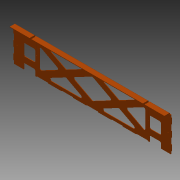
# Autodesk Inventor part: Brace
Saved by Autodesk Inventor 2014 (Build 180170000, 170)
## iProperties
Created: 2014-01-11
Part Number: Brace
Material: Aluminum 6061
Document SubType Name: Sheet Metal
Designer: Alex
Density: 2.71 g/cm^3
Sheet Metal Rule: Default
Appearance: Smooth - Light Orange
Mass: 689.694 g
Surface Area: 2287.02 cm^2
Volume: 254.5 cm^3
Author: Alex
Autodesk Inventor part; units mm, degrees
ref_plane "YZ Plane" through (0, 0, 0) normal (1, 0, 0) x (0, 1, 0)
ref_plane "XZ Plane" through (0, 0, 0) normal (0, 1, 0) x (-1, 0, 0)
ref_plane "XY Plane" through (0, 0, 0) normal (0, 0, 1) x (1, 0, 0)
sketch "Sketch1" plane through (0, 0, 0) normal (0, 0, 1) x (1, 0, 0)
  line L0 (-361.4596, 78.6852) -> (326.3724, 78.6852)
  line L1 (326.3724, -76.0008) -> (-361.4596, -76.0008)
  line L2 (328.6584, 63.6992) -> (326.3724, 63.6992)
  line L3 (326.3724, 63.6992) -> (326.3724, 38.2992)
  line L4 (326.3724, 38.2992) -> (328.6584, 38.2992)
  line L5 (328.6584, 38.2992) -> (328.6584, 63.6992)
  line L6 (326.3724, -12.5008) -> (328.6584, -12.5008)
  line L7 (328.6584, -12.5008) -> (328.6584, 12.8992)
  line L8 (328.6584, 12.8992) -> (326.3724, 12.8992)
  line L9 (326.3724, 12.8992) -> (326.3724, -12.5008)
  line L10 (328.6584, -37.9008) -> (326.3724, -37.9008)
  line L11 (326.3724, -37.9008) -> (326.3724, -63.3008)
  line L12 (326.3724, -63.3008) -> (328.6584, -63.3008)
  line L13 (328.6584, -63.3008) -> (328.6584, -37.9008)
  line L14 (-361.4596, 78.6852) -> (-361.4596, 63.6992)
  line L15 (-361.4596, 38.2992) -> (-361.4596, -76.0008)
  line L16 (326.3724, 78.6852) -> (326.3724, 63.6992)
  line L17 (326.3724, 38.2992) -> (326.3724, -76.0008)
  line L18 (328.6584, 63.6992) -> (328.6584, 38.2992)
  line L19 (328.6584, 12.8992) -> (328.6584, -12.5008)
  line L20 (328.6584, -37.9008) -> (328.6584, -63.3008)
  line L21 (-363.7456, 63.6992) -> (-361.4596, 63.6992)
  line L22 (-361.4596, 38.2992) -> (-363.7456, 38.2992)
  line L23 (-363.7456, 38.2992) -> (-363.7456, 63.6992)
  line L24 (-361.4596, -12.5008) -> (-363.7456, -12.5008)
  line L25 (-363.7456, -12.5008) -> (-363.7456, 12.8992)
  line L26 (-363.7456, 12.8992) -> (-361.4596, 12.8992)
  line L27 (-363.7456, -37.9008) -> (-361.4596, -37.9008)
  line L28 (-361.4596, -63.3008) -> (-363.7456, -63.3008)
  line L29 (-363.7456, -63.3008) -> (-363.7456, -37.9008)
  line L30 (-361.4596, -37.9008) -> (-361.4596, -63.3008)
  line L31 (-361.4596, -12.5008) -> (-361.4596, 12.8992)
  line L32 (-363.7456, 12.8992) -> (-361.4596, 12.8992)
  line L33 (-361.4596, 12.8992) -> (-361.4596, -12.5008)
  line L34 (-361.4596, -12.5008) -> (-363.7456, -12.5008)
  line L35 (-363.7456, -12.5008) -> (-363.7456, 12.8992)
  line L36 (-363.7456, -37.9008) -> (-361.4596, -37.9008)
  line L37 (-361.4596, -37.9008) -> (-361.4596, -63.3008)
  line L38 (-361.4596, -63.3008) -> (-363.7456, -63.3008)
  line L39 (-363.7456, -63.3008) -> (-363.7456, -37.9008)
  line L40 (-262.1456, 74.3672) -> (-262.1456, -76.0008)
  line L41 (227.0584, -76.0008) -> (227.0584, 76.3992)
  line L42 (-262.1456, -76.0008) -> (-211.3456, -76.0008)
  line L43 (-211.3456, -76.0008) -> (-211.3456, -73.4608)
  line L44 (-211.3456, -73.4608) -> (-262.1456, -73.4608)
  line L45 (-262.1456, -73.4608) -> (-262.1456, -76.0008)
  line L46 (-102.3161, -76.0008) -> (-102.3161, -73.4608)
  line L47 (-102.3161, -73.4608) -> (-153.1161, -73.4608)
  line L48 (-153.1161, -73.4608) -> (-153.1161, -76.0008)
  line L49 (6.7134, -76.0008) -> (6.7134, -73.4608)
  line L50 (6.7134, -73.4608) -> (-44.0866, -73.4608)
  line L51 (-44.0866, -73.4608) -> (-44.0866, -76.0008)
  line L52 (115.7429, -76.0008) -> (115.7429, -73.4608)
  line L53 (115.7429, -73.4608) -> (64.9429, -73.4608)
  line L54 (64.9429, -73.4608) -> (64.9429, -76.0008)
  line L55 (224.7723, -76.0008) -> (224.7723, -73.4608)
  line L56 (224.7723, -73.4608) -> (173.9723, -73.4608)
  line L57 (173.9723, -73.4608) -> (173.9723, -76.0008)
  line L58 (-153.1161, -76.0008) -> (-102.3161, -76.0008)
  line L59 (-44.0866, -76.0008) -> (6.7134, -76.0008)
  line L60 (64.9429, -76.0008) -> (115.7429, -76.0008)
  line L61 (173.9723, -76.0008) -> (224.7723, -76.0008)
  line L62 (-361.4596, 78.6852) -> (-356.3796, 78.6852)
  line L63 (-356.3796, 78.6852) -> (-356.3796, 74.1132)
  line L64 (-356.3796, 74.1132) -> (-361.4596, 74.1132)
  line L65 (-361.4596, 74.1132) -> (-361.4596, 78.6852)
  line L66 (326.3724, 78.6852) -> (321.2924, 78.6852)
  line L67 (321.2924, 78.6852) -> (321.2924, 74.1132)
  line L68 (321.2924, 74.1132) -> (326.3724, 74.1132)
  line L69 (326.3724, 74.1132) -> (326.3724, 78.6852)
  point P0 (0, 0)
  point P1 (-362.6026, 63.6992)
  dimension "d0" = 687.832
  dimension "d3" = 2.286
  dimension "d4" = 25.4
  dimension "d5" = 14.986
  dimension "d6" = 25.4
  dimension "d7" = 2.286
  dimension "d8" = 25.4
  dimension "d9" = 2.286
  dimension "d10" = 25.4
  dimension "d11" = 25.4
  dimension "d12" = 2.286
  dimension "d13" = 2.286
  dimension "d16" = 50.8
  dimension "d17" = 2.54
  dimension "d21" = 109.0295
  dimension "d84" = 5.08
  dimension "d85" = 5.08
  dimension "d90" = 4.572
  dimension "d91" = 4.572
  measures "d0" distance of L1.start L1.end
  measures "d3" distance of L4.end L3.end
  measures "d4" distance of L3.end L2.end
  measures "d5" distance between parallel lines of L0 L2
  measures "d6" distance of L8.end L6.start
  measures "d7" distance of L7.end L8.end
  measures "d8" distance from line of L3.end L8
  measures "d9" distance of L12.end L11.end
  measures "d10" distance of L11.end L10.end
  measures "d11" distance between parallel lines of L6 L10
  measures "d12" distance of L24.start L25.start
  measures "d13" distance of L15.start L23.start
  measures "d16" distance of L44.end L43.end
  measures "d17" distance of L43.end L42.end
  measures "d21" distance of L44.end L48.start
  measures "d84" distance of L63.end L64.end
  measures "d85" distance of L68.end L67.end
  measures "d90" distance between parallel lines of L62 L64
  measures "d91" distance between parallel lines of L0 L68
extrude "Plate1" add sketch "Sketch1" along normal blind 2.286 contours L0 L67 L68 L16 L3 L17 L9 L11 L1 L55 L56 L57 L52 L53 L54 L49 L50 L51 L46 L47 L48 L43 L44 L40 L15 L22 L23 L21 L14 L64 L63 | L2 L5 L4 L3 | L15 L24 L25 L26 | L8 L7 L6 L9 | L15 L28 L29 L27 | L10 L13 L12 L11
sketch "Sketch3" plane through (0, 0, 2.286) normal (0, 0, 1) x (1, 0, 0)
  line L0 (328.6584, 12.8992) -> (328.6584, -12.5008) projected
  line L1 (-356.3796, 78.6852) -> (321.2924, 78.6852) projected
  line L2 (-363.7456, -12.5008) -> (-363.7456, 12.8992) projected
  line L3 (-264.4316, 78.6852) -> (-262.1456, 78.6852)
  line L4 (-262.1456, 78.6852) -> (-262.1456, 2.4852)
  line L5 (-262.1456, 2.4852) -> (-264.4316, 2.4852)
  line L6 (-264.4316, 2.4852) -> (-264.4316, 78.6852)
  line L7 (227.0584, 78.6852) -> (229.3444, 78.6852)
  line L8 (229.3444, 78.6852) -> (229.3444, 2.4852)
  line L9 (229.3444, 2.4852) -> (227.0584, 2.4852)
  line L10 (227.0584, 2.4852) -> (227.0584, 78.6852)
  line L11 (-264.4316, 78.6852) -> (-269.5116, 78.6852)
  line L12 (-269.5116, 78.6852) -> (-269.5116, 74.1132)
  line L13 (-269.5116, 74.1132) -> (-264.4316, 74.1132)
  line L14 (-264.4316, 74.1132) -> (-264.4316, 78.6852)
  line L15 (229.3444, 78.6852) -> (234.4244, 78.6852)
  line L16 (234.4244, 78.6852) -> (234.4244, 74.1132)
  line L17 (234.4244, 74.1132) -> (229.3444, 74.1132)
  line L18 (229.3444, 74.1132) -> (229.3444, 78.6852)
  point P0 (326.3724, 78.6852)
  point P1 (-361.4596, 78.6852)
  point P2 (0, 0)
  dimension "d26" = 2.286
  dimension "d27" = 76.2
  dimension "d28" = 101.6
  dimension "d29" = 2.286
  dimension "d30" = 76.2
  dimension "d31" = 101.6
  dimension "d86" = 5.08
  dimension "d87" = 5.08
  dimension "d88" = 4.572
  dimension "d89" = 4.572
  constraints: 32 end point, 8 parallel, 4 horizontal, 4 perpendicular, 2 point on line
  measures "d26" distance of L4.end L5.end
  measures "d27" distance of L3.end L4.end
  measures "d28" distance between parallel lines of L2 L4
  measures "d29" distance of L8.end L9.end
  measures "d30" distance of L7.end L8.end
  measures "d31" distance between parallel lines of L0 L10
  measures "d86" distance of L13.end L12.end
  measures "d87" distance of L16.end L17.end
  measures "d88" distance between parallel lines of L1 L13
  measures "d89" distance between parallel lines of L1 L17
extrude "Cut2" cut sketch "Sketch3" against normal blind 2.286
sketch "Sketch4" plane through (0, 0, 2.286) normal (0, 0, 1) x (1, 0, 0)
  line L0 (229.3444, 74.1132) -> (229.3444, 2.4852) projected
  line L1 (-264.4316, 2.4852) -> (-264.4316, 74.1132) projected
  line L2 (-262.1456, -76.0008) -> (-361.4596, -76.0008) projected
  line L3 (326.3724, -76.0008) -> (224.7723, -76.0008) projected
  line L4 (-267.6066, -76.0008) -> (-318.4066, -76.0008)
  line L5 (-318.4066, -76.0008) -> (-318.4066, 25.5992)
  line L6 (-318.4066, 25.5992) -> (-267.6066, 25.5992)
  line L7 (-267.6066, 25.5992) -> (-267.6066, -76.0008)
  line L8 (283.3194, -76.0008) -> (232.5194, -76.0008)
  line L9 (232.5194, -76.0008) -> (232.5194, 25.5992)
  line L10 (232.5194, 25.5992) -> (283.3194, 25.5992)
  line L11 (283.3194, 25.5992) -> (283.3194, -76.0008)
  point P0 (229.3444, 78.6852)
  point P1 (-264.4316, 78.6852)
  point P2 (0, 0)
  dimension "d34" = 50.8
  dimension "d35" = 101.6
  dimension "d37" = 3.175
  dimension "d38" = 50.8
  dimension "d40" = 3.175
  dimension "d41" = 101.6
  constraints: 16 end point, 4 parallel, 2 collinear, 2 horizontal, 2 perpendicular
  measures "d34" distance of L5.end L6.end
  measures "d35" distance between parallel lines of L6 L4
  measures "d37" distance between parallel lines of L7 L1
  measures "d38" distance of L9.end L10.end
  measures "d40" distance between parallel lines of L0 L9
  measures "d41" distance between parallel lines of L10 L8
extrude "Cut3" cut sketch "Sketch4" against normal blind 2.286
fillet "Corner Round1" radius 6.35 4 edges at (-318.4066, 25.5992, 1.143) (-267.6066, 25.5992, 1.143) (283.3194, 25.5992, 1.143) (232.5194, 25.5992, 1.143)
sketch "Sketch5" plane through (0, 0, 2.286) normal (0, 0, 1) x (1, 0, 0)
  line L0 (-267.6066, 19.2492) -> (-267.6066, -76.0008) projected
  arc A0 (-277.1316, -37.9008) -> (-270.7816, -31.5508) centre (-277.1316, -31.5508) ccw projected
  line L1 (-277.1316, -37.9008) -> (-340.6316, -37.9008) projected
  arc A1 (-346.9816, -31.5508) -> (-340.6316, -37.9008) centre (-340.6316, -31.5508) ccw projected
  line L2 (-318.4066, -76.0008) -> (-318.4066, 19.2492) projected
  arc A2 (-312.0566, 25.5992) -> (-318.4066, 19.2492) centre (-312.0566, 19.2492) ccw projected
  line L3 (-312.0566, 25.5992) -> (-273.9566, 25.5992) projected
  arc A3 (-267.6066, 19.2492) -> (-273.9566, 25.5992) centre (-273.9566, 19.2492) ccw projected
  line L4 (283.3194, 19.2492) -> (283.3194, -76.0008) projected
  arc A4 (305.5444, -37.9008) -> (311.8944, -31.5508) centre (305.5444, -31.5508) ccw projected
  line L5 (305.5444, -37.9008) -> (242.0444, -37.9008) projected
  arc A5 (235.6944, -31.5508) -> (242.0444, -37.9008) centre (242.0444, -31.5508) ccw projected
  line L6 (232.5194, -76.0008) -> (232.5194, 19.2492) projected
  arc A6 (238.8694, 25.5992) -> (232.5194, 19.2492) centre (238.8694, 19.2492) ccw projected
  line L7 (238.8694, 25.5992) -> (276.9694, 25.5992) projected
  arc A7 (283.3194, 19.2492) -> (276.9694, 25.5992) centre (276.9694, 19.2492) ccw projected
  line L8 (229.3444, 74.1132) -> (229.3444, 2.4852) projected
  line L9 (229.3444, 2.4852) -> (227.0584, 2.4852) projected
  line L10 (227.0584, 2.4852) -> (227.0584, 78.6852) projected
  line L11 (-262.1456, 78.6852) -> (227.0584, 78.6852) projected
  line L12 (-262.1456, 78.6852) -> (-262.1456, 2.4852) projected
  line L13 (-262.1456, 2.4852) -> (-264.4316, 2.4852) projected
  line L14 (-264.4316, 2.4852) -> (-264.4316, 74.1132) projected
  line L15 (-356.3796, 78.6852) -> (-269.5116, 78.6852) projected
  line L16 (-361.4596, 63.6992) -> (-361.4596, 74.1132) projected
  line L17 (-363.7456, 63.6992) -> (-361.4596, 63.6992) projected
  line L18 (-363.7456, 38.2992) -> (-363.7456, 63.6992) projected
  line L19 (-361.4596, 38.2992) -> (-363.7456, 38.2992) projected
  line L20 (-361.4596, 12.8992) -> (-361.4596, 38.2992) projected
  line L21 (-363.7456, 12.8992) -> (-361.4596, 12.8992) projected
  line L22 (-363.7456, -12.5008) -> (-363.7456, 12.8992) projected
  line L23 (-361.4596, -12.5008) -> (-363.7456, -12.5008) projected
  line L24 (-361.4596, -37.9008) -> (-361.4596, -12.5008) projected
  line L25 (-363.7456, -37.9008) -> (-361.4596, -37.9008) projected
  line L26 (-363.7456, -63.3008) -> (-363.7456, -37.9008) projected
  line L27 (-361.4596, -63.3008) -> (-363.7456, -63.3008) projected
  line L28 (-361.4596, -76.0008) -> (-361.4596, -63.3008) projected
  line L29 (-262.1456, -76.0008) -> (-361.4596, -76.0008) projected
  line L30 (-262.1456, -76.0008) -> (-262.1456, -73.4608) projected
  line L31 (-262.1456, -73.4608) -> (-211.3456, -73.4608) projected
  line L32 (-211.3456, -73.4608) -> (-211.3456, -76.0008) projected
  line L33 (-153.1161, -76.0008) -> (-211.3456, -76.0008) projected
  line L34 (-153.1161, -76.0008) -> (-153.1161, -73.4608) projected
  line L35 (-153.1161, -73.4608) -> (-102.3161, -73.4608) projected
  line L36 (-102.3161, -73.4608) -> (-102.3161, -76.0008) projected
  line L37 (-44.0866, -76.0008) -> (-102.3161, -76.0008) projected
  line L38 (-44.0866, -76.0008) -> (-44.0866, -73.4608) projected
  line L39 (-44.0866, -73.4608) -> (6.7134, -73.4608) projected
  line L40 (6.7134, -73.4608) -> (6.7134, -76.0008) projected
  line L41 (64.9429, -76.0008) -> (6.7134, -76.0008) projected
  line L42 (64.9429, -76.0008) -> (64.9429, -73.4608) projected
  line L43 (64.9429, -73.4608) -> (115.7429, -73.4608) projected
  line L44 (115.7429, -73.4608) -> (115.7429, -76.0008) projected
  line L45 (173.9723, -76.0008) -> (115.7429, -76.0008) projected
  line L46 (173.9723, -76.0008) -> (173.9723, -73.4608) projected
  line L47 (173.9723, -73.4608) -> (224.7723, -73.4608) projected
  line L48 (224.7723, -73.4608) -> (224.7723, -76.0008) projected
  line L49 (326.3724, -76.0008) -> (224.7723, -76.0008) projected
  line L50 (326.3724, -63.3008) -> (326.3724, -76.0008) projected
  line L51 (328.6584, -63.3008) -> (326.3724, -63.3008) projected
  line L52 (328.6584, -37.9008) -> (328.6584, -63.3008) projected
  line L53 (326.3724, -37.9008) -> (328.6584, -37.9008) projected
  line L54 (326.3724, -12.5008) -> (326.3724, -37.9008) projected
  line L55 (328.6584, -12.5008) -> (326.3724, -12.5008) projected
  line L56 (328.6584, 12.8992) -> (328.6584, -12.5008) projected
  line L57 (326.3724, 12.8992) -> (328.6584, 12.8992) projected
  line L58 (326.3724, 38.2992) -> (326.3724, 12.8992) projected
  line L59 (328.6584, 38.2992) -> (326.3724, 38.2992) projected
  line L60 (328.6584, 63.6992) -> (328.6584, 38.2992) projected
  line L61 (326.3724, 63.6992) -> (328.6584, 63.6992) projected
  line L62 (326.3724, -63.3008) -> (326.3724, 63.6992) projected
  line L63 (-356.3796, 78.6852) -> (-269.5116, 78.6852) projected
  point P0 (229.3444, 78.6852)
  point P1 (-264.4316, 78.6852)
  point P2 (-361.4596, 78.6852)
  point P3 (326.3724, 78.6852)
  point P4 (0, 0)
  constraints: 4 other
sketch "Sketch6" plane through (-262.1456, 76.3992, 0) normal (0, 1, 0) x (-1, 0, 0)
  line L0 (-489.204, 0) -> (0, 0)
  line L1 (0, 0) -> (0, 25.4)
  line L2 (0, 25.4) -> (-489.204, 25.4)
  line L3 (-489.204, 25.4) -> (-489.204, 0)
  constraints: 6 end point, 1 horizontal, 1 perpendicular, 1 vertical
edge flange "Flange1" height 25.4 angle 90 thickness 2.286 bend radius 2.286 thickness toward (0, 1, 0) relief straight relief width 2.286 relief depth 1.143 corner gap 2.286 corner form 0 edges at (-17.5436, 78.6852, 2.286) (277.8584, 78.6852, 2.286) (-312.9456, 78.6852, 2.286) wall of the first edge with corners at (227.0584, 76.3992, 0) (-262.1456, 76.3992, 0) (-262.1456, 76.3992, 25.4) (227.0584, 76.3992, 25.4)
bend "Bend1"
corner "Corner1"
sketch "Sketch7" plane through (0, 0, 2.286) normal (0, 0, 1) x (1, 0, 0)
  line L0 (-318.4066, -76.0008) -> (-361.4596, -76.0008)
  line L1 (-318.4066, -76.0008) -> (-318.4066, 19.2492)
  line L2 (-267.6066, 19.2492) -> (-267.6066, -76.0008)
  line L3 (232.5194, -76.0008) -> (224.7723, -76.0008)
  line L4 (232.5194, -76.0008) -> (232.5194, 19.2492)
  line L5 (283.3194, 19.2492) -> (283.3194, -76.0008)
  line L6 (232.5194, -25.2008) -> (283.3194, -25.2008)
  line L7 (283.3194, -25.2008) -> (283.3194, -50.6008)
  line L8 (283.3194, -50.6008) -> (232.5194, -50.6008)
  line L9 (232.5194, -50.6008) -> (232.5194, -25.2008)
  line L10 (-267.6066, -50.6008) -> (-318.4066, -50.6008)
  line L11 (-318.4066, -50.6008) -> (-318.4066, -25.2008)
  line L12 (-318.4066, -25.2008) -> (-267.6066, -25.2008)
  line L13 (-267.6066, -25.2008) -> (-267.6066, -50.6008)
  point P0 (0, 0)
  dimension "d55" = 25.4
  dimension "d56" = 25.4
  dimension "d57" = 25.4
  dimension "d58" = 25.4
  measures "d55" distance between parallel lines of L8 L3
  measures "d56" distance between parallel lines of L8 L6
  measures "d57" distance between parallel lines of L10 L0
  measures "d58" distance between parallel lines of L10 L12
sheet face with bend "Face2" sketch "Sketch7" thickness 2.286 toward (0, 0, -1) bend radius 2.286 relief straight relief width 2.286 relief depth 1.143
bend "Bend2"
fillet "Corner Round2" radius 6.35 8 edges at (-318.4066, -25.2008, 1.143) (-267.6066, -25.2008, 1.143) (283.3194, -25.2008, 1.143) (232.5194, -25.2008, 1.143) (283.3194, -50.6008, 1.143) (232.5194, -50.6008, 1.143) (-318.4066, -50.6008, 1.143) (-267.6066, -50.6008, 1.143)
sketch "Sketch8" plane through (0, 0, 2.286) normal (0, 0, 1) x (1, 0, 0)
  line L0 (227.0584, 2.4852) -> (227.0584, 74.1132) projected
  line L1 (227.0584, 74.1132) -> (-262.1456, 74.1132) projected
  line L2 (-262.1456, 74.1132) -> (-262.1456, 2.4852) projected
  line L3 (64.9429, -73.4608) -> (115.7429, -73.4608) projected
  line L4 (-249.4456, 61.4132) -> (214.3584, 61.4132)
  line L5 (214.3584, 61.4132) -> (214.3584, -60.7608)
  line L6 (214.3584, -60.7608) -> (-249.4456, -60.7608)
  line L7 (-249.4456, -60.7608) -> (-249.4456, 61.4132)
  line L8 (-17.5436, 61.4132) -> (214.3584, -60.7608)
  line L9 (214.3584, 61.4132) -> (-17.5436, -60.7608)
  line L10 (-249.4456, 61.4132) -> (-17.5436, -60.7608)
  line L11 (-17.5436, 61.4132) -> (-249.4456, -60.7608)
  line L12 (-222.1985, -60.7608) -> (-119.871, -6.8512)
  line L13 (-17.5436, -60.7608) -> (-133.4946, 0.3262)
  line L14 (-44.7906, -60.7608) -> (-147.1181, -6.8512)
  line L15 (-147.1181, -6.8512) -> (-249.4456, 47.0585)
  line L16 (-249.4456, -46.4061) -> (-133.4946, 14.6809)
  line L17 (9.7035, -60.7608) -> (-222.1985, 61.4132)
  line L18 (-119.871, -6.8512) -> (9.7035, 61.4132)
  line L19 (187.1114, -60.7608) -> (-31.1671, 54.2358)
  line L20 (214.3584, -46.4061) -> (9.7035, 61.4132)
  line L21 (217.3789, 48.6498) -> (9.7035, -60.7608)
  line L22 (187.1114, 61.4132) -> (-44.7906, -60.7608)
  line L23 (-222.1985, 61.4132) -> (-133.4946, 14.6809)
  line L24 (-133.4946, 14.6809) -> (-88.6639, 38.2992)
  line L25 (-44.7906, 61.4132) -> (-222.1985, 61.4132)
  line L26 (-249.4456, 47.0585) -> (-160.7416, 0.3262)
  line L27 (-160.7416, 0.3262) -> (-249.4456, -46.4061)
  line L28 (-222.1985, -60.7608) -> (-133.4946, -14.0285)
  line L29 (-133.4946, -14.0285) -> (-44.7906, -60.7608)
  line L30 (-44.7906, -60.7608) -> (-222.1985, -60.7608)
  line L31 (-17.5436, -46.4061) -> (71.1604, 0.3262)
  line L32 (71.1604, 0.3262) -> (-17.5436, 47.0585)
  line L33 (-106.2475, 0.3262) -> (-17.5436, 47.0585)
  line L34 (-106.2475, 0.3262) -> (-17.5436, -46.4061)
  line L35 (9.7035, -60.7608) -> (98.4074, -14.0285)
  line L36 (187.1114, -60.7608) -> (98.4074, -14.0285)
  line L37 (187.1114, -60.7608) -> (9.7035, -60.7608)
  line L38 (125.6545, 0.3262) -> (214.3584, -46.4061)
  line L39 (187.1114, 61.4132) -> (98.4074, 14.6809)
  line L40 (98.4074, 14.6809) -> (9.7035, 61.4132)
  line L41 (-44.7906, 61.4132) -> (-222.1985, 61.4132)
  line L42 (-88.6639, 38.2992) -> (-133.4946, 14.6809)
  line L43 (-133.4946, 14.6809) -> (-222.1985, 61.4132)
  line L44 (232.5194, -76.0008) -> (232.5194, -56.9508) projected
  line L45 (9.7035, 61.4132) -> (98.4074, 14.6809)
  line L46 (98.4074, 14.6809) -> (187.1114, 61.4132)
  line L47 (187.1114, 61.4132) -> (9.7035, 61.4132)
  line L48 (214.3584, 47.0585) -> (125.6545, 0.3262)
  line L49 (125.6545, 0.3262) -> (214.3584, -46.4061)
  line L50 (214.3584, -46.4061) -> (214.3584, 47.0585)
  line L51 (232.5194, -76.0008) -> (224.7723, -76.0008) projected
  line L52 (-133.4946, -14.0285) -> (-44.7906, -60.7608)
  line L53 (-44.7906, -60.7608) -> (-222.1985, -60.7608)
  line L54 (-222.1985, -60.7608) -> (-133.4946, -14.0285)
  line L55 (-133.4946, 14.6809) -> (-88.6639, 38.2992)
  line L56 (-44.7906, 61.4132) -> (-222.1985, 61.4132)
  line L57 (-222.1985, 61.4132) -> (-133.4946, 14.6809)
  line L58 (-361.4596, 38.2992) -> (-363.7456, 38.2992) projected
  line L59 (-133.4946, 14.6809) -> (-44.7906, 61.4132)
  line L60 (-44.7906, 61.4132) -> (-222.1985, 61.4132)
  point P0 (0, 0)
  point P1 (227.0584, 78.6852)
  point P2 (-262.1456, 78.6852)
  dimension "d65" = 12.7
  dimension "d66" = 12.7
  dimension "d67" = 12.7
  dimension "d68" = 12.7
  dimension "d69" = 12.7
  dimension "d71" = 231.902
  dimension "d72" = 463.804
  dimension "d73" = 231.902
  dimension "d74" = 12.7
  dimension "d75" = 12.7
  dimension "d76" = 12.7
  dimension "d77" = 12.7
  dimension "d78" = 12.7
  dimension "d79" = 12.7
  constraints: 106 end point, 30 point on line, 13 parallel, 10 collinear, 4 midpoint, 3 horizontal, 2 perpendicular, 11 other
  measures "d65" distance between parallel lines of L2 L7
  measures "d66" distance between parallel lines of L1 L4
  measures "d67" distance between parallel lines of L5 L0
  measures "d69" distance between parallel lines of L11 L12
  measures "d71" distance of L7.start L9.end
  measures "d72" distance between parallel lines of L5 L7
  measures "d73" distance of L4.start L8.start
  measures "d74" distance between parallel lines of L14 L13
  measures "d75" distance between parallel lines of L11 L16
  measures "d76" distance between parallel lines of L10 L17
  measures "d77" distance between parallel lines of L8 L19
  measures "d78" distance between parallel lines of L9 L21
  measures "d79" distance between parallel lines of L9 L22
extrude "Cut4" cut sketch "Sketch8" against normal blind 2.286 contours L4 L59 L24 L17 | L15 L16 L7 | L4 L22 L20 | L18 L19 L22 L17 | L12 L14 L6 | L21 L19 L6 | L5 L20 L21
fillet "Corner Round3" radius 6.35 13 edges at (-17.5436, -46.4061, 1.143) (71.1604, 0.3262, 1.143) (98.4074, 14.6809, 1.143) (98.4074, -14.0285, 1.143) (125.6545, 0.3262, 1.143) (187.1114, -60.7608, 1.143) (9.7035, -60.7608, 1.143) (-222.1985, -60.7608, 1.143) (-160.7416, 0.3262, 1.143) (-249.4456, 47.0585, 1.143) (-222.1985, 61.4132, 1.143) (9.7035, 61.4132, 1.143) (-44.7906, 61.4132, 1.143)
fillet "Corner Round4" radius 6.35 9 edges at (-106.2475, 0.3262, 1.143) (-133.4946, -14.0285, 1.143) (-249.4456, -46.4061, 1.143) (-133.4946, 14.6809, 1.143) (-17.5436, 47.0585, 1.143) (187.1114, 61.4132, 1.143) (214.3584, 47.0585, 1.143) (214.3584, -46.4061, 1.143) (-44.7906, -60.7608, 1.143)
sketch "Sketch9" plane through (0, 0, 2.286) normal (0, 0, 1) x (1, 0, 0)
  line L0 (326.3724, 38.2992) -> (326.3724, 12.8992) projected
  line L1 (227.0584, 2.4852) -> (227.0584, 74.1132) projected
  line L2 (227.0584, 74.1132) -> (-262.1456, 74.1132) projected
  line L3 (-262.1456, 74.1132) -> (-262.1456, 2.4852) projected
  line L4 (-361.4596, 12.8992) -> (-361.4596, 38.2992) projected
  circle A0 centre (-348.5056, 0) radius 1.5875
  circle A1 centre (-249.1916, 61.4132) radius 1.5875
  circle A2 centre (214.1044, 61.4132) radius 1.5875
  circle A3 centre (313.4184, 0) radius 1.5875
  point P0 (0, 0)
  dimension "d92" = 3.175
  dimension "d93" = 12.954
  dimension "d94" = 3.175
  dimension "d95" = 12.954
  dimension "d96" = 12.7
  dimension "d97" = 3.175
  dimension "d98" = 12.954
  dimension "d99" = 12.7
  dimension "d100" = 3.175
  dimension "d101" = 12.954
  constraints: 4 centre point
  measures "d92" diameter of A0
  measures "d93" distance from line of L4 A0.centre
  measures "d94" diameter of A1
  measures "d95" distance from line of L3 A1.centre
  measures "d96" distance from line of L2 A1.centre
  measures "d97" diameter of A2
  measures "d98" distance from line of L1 A2.centre
  measures "d99" distance from line of L2 A2.centre
  measures "d100" diameter of A3
  measures "d101" distance from line of L0 A3.centre
extrude "Cut5" cut sketch "Sketch9" against normal blind 2.286
sketch "Sketch10" plane through (0, 0, 2.286) normal (0, 0, 1) x (1, 0, 0)
  line L0 (-44.0866, -73.4608) -> (6.7134, -73.4608) projected
  circle A0 centre (-17.5436, -60.5068) radius 1.5875
  point P0 (0, 0)
  dimension "d104" = 3.175
  dimension "d105" = 12.954
  constraints: 1 centre point
  measures "d104" diameter of A0
  measures "d105" distance from line of L0 A0.centre
extrude "Cut6" cut sketch "Sketch10" against normal blind 2.286
equation "\"d32\" = Thickness"
equation "\"d42\" = Thickness"
equation "\"d65\" = d68"
equation "\"d66\" = d65"
equation "\"d67\" = d68"
equation "\"d71\" = 0.5 * d72"
equation "\"d73\" = d71"
equation "\"d80\" = Thickness"
equation "\"d45\" = BendReliefWidth"
equation "\"d46\" = BendReliefDepth"
equation "\"d47\" = MinimumRemnant"
equation "\"d48\" = BendRadius"
equation "\"d51\" = BendRadius"
equation "\"d52\" = CornerReliefSize"
equation "\"d53\" = GapSize"
equation "\"d54\" = JacobiRadiusSize"
equation "\"d59\" = BendRadius"
equation "\"d60\" = BendReliefWidth"
equation "\"d62\" = MinimumRemnant"
equation "\"d61\" = BendReliefDepth"
equation "\"d63\" = BendRadius"
equation "\"BendRadius\" = Thickness"
equation "\"BendReliefWidth\" = Thickness"
equation "\"BendReliefDepth\" = 0.5 * Thickness"
equation "\"CornerReliefSize\" = 4 * Thickness"
equation "\"MinimumRemnant\" = 2 * Thickness"
equation "\"TransitionRadius\" = BendRadius"
equation "\"JacobiRadiusSize\" = BendRadius"
equation "\"GapSize\" = Thickness"
equation "\"d2\" = BendRadius"
equation "\"Thickness\" = 2.286"
body "Solid1"
